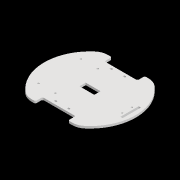
# Autodesk Inventor part: Parte inferior 2 v1
Saved by Autodesk Inventor 2022 (Build 260153000, 153)
## iProperties
Created: 2021-09-27
Part Number: Parte inferior 2 v1
Material: Genérico
Document SubType Name: Modeling
Designer: Julio R
Density: 1 g/cm^3
Appearance: Valor por defecto
Author: Julio R
Autodesk Inventor part; units mm, degrees
ref_plane "YZ Plane" through (0, 0, 0) normal (1, 0, 0) x (0, 1, 0)
ref_plane "XZ Plane" through (0, 0, 0) normal (0, 1, 0) x (-1, 0, 0)
ref_plane "XY Plane" through (0, 0, 0) normal (0, 0, 1) x (1, 0, 0)
sketch "Boceto2" plane through (0, 0, 0) normal (0, 1, 0) x (-1, 0, 0)
  circle A0 centre (0, 0) radius 62.5
  line L0 (15, 32.5) -> (15, -32.5)
  line L1 (15, -32.5) -> (45, -32.5)
  line L2 (45, -32.5) -> (45, 32.5)
  line L3 (45, 32.5) -> (15, 32.5)
  circle A1 centre (18.5, -29) radius 1.25
  line L4 (0, 6.809) -> (0, -6.809)
  line L5 (-6.4675, 0) -> (6.4675, 0) construction
  circle A2 centre (41.5, -29) radius 1.25
  circle A3 centre (18.5, 29) radius 1.25
  circle A4 centre (41.5, 29) radius 1.25
  line L6 (7.5, -42.3) -> (-7.5, -42.3)
  line L7 (-7.5, -42.3) -> (-7.5, -25)
  line L8 (-7.5, -25) -> (7.5, -25)
  line L9 (7.5, -25) -> (7.5, -42.3)
  arc A5 (9, -42.3) -> (9, -33.8) centre (9, -38.05) ccw
  line L10 (9, -42.3) -> (7.5, -42.3)
  line L11 (9, -33.8) -> (7.5, -33.8)
  arc A6 (9.5, -39.2) -> (9.5, -36.9) centre (9.5, -38.05) ccw
  line L12 (9.5, -39.2) -> (7.5, -39.2)
  line L13 (7.5, -39.2) -> (7.5, -36.9)
  line L14 (7.5, -36.9) -> (9.5, -36.9)
  line L15 (9.5, -36.9) -> (9.5, -39.2)
  arc A7 (-9, -33.8) -> (-9, -42.3) centre (-9, -38.05) ccw
  line L16 (-9, -42.3) -> (-7.5, -42.3)
  line L17 (-9, -33.8) -> (-7.5, -33.8)
  arc A8 (-9.5, -36.9) -> (-9.5, -39.2) centre (-9.5, -38.05) ccw
  line L18 (-9.5, -39.2) -> (-7.5, -39.2)
  line L19 (-7.5, -39.2) -> (-7.5, -36.9)
  line L20 (-7.5, -36.9) -> (-9.5, -36.9)
  line L21 (-9.5, -36.9) -> (-9.5, -39.2)
  line L22 (7.5, 42.3) -> (-7.5, 42.3)
  line L23 (-7.5, 42.3) -> (-7.5, 25)
  line L24 (-7.5, 25) -> (7.5, 25)
  line L25 (7.5, 25) -> (7.5, 42.3)
  arc A9 (9, 33.8) -> (9, 42.3) centre (9, 38.05) ccw
  line L26 (9, 42.3) -> (7.5, 42.3)
  line L27 (9, 33.8) -> (7.5, 33.8)
  arc A10 (9.5, 36.9) -> (9.5, 39.2) centre (9.5, 38.05) ccw
  line L28 (9.5, 39.2) -> (7.5, 39.2)
  line L29 (7.5, 39.2) -> (7.5, 36.9)
  line L30 (7.5, 36.9) -> (9.5, 36.9)
  line L31 (9.5, 36.9) -> (9.5, 39.2)
  line L32 (-9, 33.8) -> (-7.5, 33.8)
  line L33 (-7.5, 36.9) -> (-9.5, 36.9)
  line L34 (-7.5, 39.2) -> (-7.5, 36.9)
  line L35 (-9.5, 36.9) -> (-9.5, 39.2)
  line L36 (-9.5, 39.2) -> (-7.5, 39.2)
  arc A11 (-9.5, 39.2) -> (-9.5, 36.9) centre (-9.5, 38.05) ccw
  line L37 (-9, 42.3) -> (-7.5, 42.3)
  arc A12 (-9, 42.3) -> (-9, 33.8) centre (-9, 38.05) ccw
  line L38 (-15, -31) -> (-48, -31)
  line L39 (-48, -31) -> (-48, 31)
  line L40 (-48, 31) -> (-15, 31)
  line L41 (-15, 31) -> (-15, -31)
  line L42 (10.1, -4.25) -> (-10.1, -4.25)
  line L43 (-10.1, -4.25) -> (-10.1, 4.25)
  line L44 (-10.1, 4.25) -> (10.1, 4.25)
  line L45 (10.1, 4.25) -> (10.1, -4.25)
  line L46 (46.0104, -42.3) -> (-46.0104, -42.3)
  line L47 (-46.0104, -42.3) -> (-46.0104, 42.3)
  line L48 (-46.0104, 42.3) -> (46.0104, 42.3)
  line L49 (46.0104, 42.3) -> (46.0104, -42.3)
  line L50 (-54, -12.5) -> (-57, -12.5)
  line L51 (-57, -12.5) -> (-57, 12.5)
  line L52 (-57, 12.5) -> (-54, 12.5)
  line L53 (-54, 12.5) -> (-54, -12.5)
  line L54 (58.7, -12.5) -> (46, -12.5)
  line L55 (46, -12.5) -> (46, 7.82)
  line L56 (46, 7.82) -> (58.7, 7.82)
  line L57 (58.7, 7.82) -> (58.7, -12.5)
  line L58 (22.5, 52.3) -> (-22.5, 52.3)
  line L59 (-22.5, 52.3) -> (-22.5, 42.3)
  line L60 (-22.5, 42.3) -> (22.5, 42.3)
  line L61 (22.5, 42.3) -> (22.5, 52.3)
  line L62 (22.5, -52.3) -> (-22.5, -52.3)
  line L63 (-22.5, -52.3) -> (-22.5, -42.3)
  line L64 (-22.5, -42.3) -> (22.5, -42.3)
  line L65 (22.5, -42.3) -> (22.5, -52.3)
  line L66 (22.5, 52.3) -> (34.2193, 52.3)
  line L67 (-22.5, 52.3) -> (-34.2193, 52.3)
  line L68 (22.5, -52.3) -> (34.2193, -52.3)
  line L69 (-22.5, -52.3) -> (-34.2193, -52.3)
  circle A13 centre (-50.6, 6.809) radius 1.15
  circle A14 centre (-50.6, -6.653) radius 1.15
  point P0 (45, 0)
  point P1 (13.25, -38.05)
  point P2 (10.65, -38.05)
  point P3 (-13.25, -38.05)
  point P4 (-10.65, -38.05)
  point P5 (13.25, 38.05)
  point P6 (10.65, 38.05)
  point P7 (-10.65, 38.05)
  point P8 (-13.25, 38.05)
  point P9 (-15, 0)
  point P10 (0, -4.25)
  point P11 (10.1, 0)
  point P12 (-54, 0)
  point P13 (9, 42.3)
  point P14 (0, 52.3)
  point P15 (-22.5, -42.3)
  point P16 (22.5, -42.3)
  point P17 (22.5, 42.3)
  dimension "d51" = 125
  dimension "d52" = 65
  dimension "d53" = 30
  dimension "d56" = 3.5
  dimension "d57" = 3.5
  dimension "d60" = 23
  dimension "d63" = 58
  dimension "d70" = 15
  dimension "d78" = 15
  dimension "d79" = 17.3
  dimension "d80" = 8.5
  dimension "d81" = 1.5
  dimension "d82" = 4.25
  dimension "d83" = 1.15
  dimension "d84" = 2.3
  dimension "d86" = 2
  dimension "d87" = 25
  dimension "d88" = 7.5
  dimension "d89" = 33
  dimension "d90" = 62
  dimension "d91" = 15
  dimension "d92" = 20.2
  dimension "d93" = 8.5
  dimension "d94" = 3
  dimension "d95" = 25
  dimension "d98" = 6
  dimension "d99" = 12.7
  dimension "d100" = 20.32
  dimension "d101" = 1
  dimension "d102" = 20
  dimension "d108" = 10
  dimension "d113" = 45
  dimension "d114" = 13.462
  dimension "d115" = 3.4
  dimension "d116" = 2.3
  dimension "d119" = 2.3
  constraints: 140 end point, 41 symmetric about line, 24 point on circle, 20 parallel, 15 centre point, 13 horizontal, 9 perpendicular, 8 midpoint, 5 horizontal alignment, 4 coincident, 4 collinear, 4 point on line, 4 vertical alignment, 2 vertical, 12 other
  measures "d51" diameter of A0
  measures "d52" distance of L2.end L1.end
  measures "d53" distance of L1.end L0.end
  measures "d56" horizontal distance of A1.centre L0.end
  measures "d57" horizontal distance of L0.end A1.centre
  measures "d60" distance of A1.centre A2.centre
  measures "d63" distance of A1.centre A3.centre
  measures "d70" distance from line of point (0, 0) L0
  measures "d78" distance of L7.end L8.end
  measures "d79" distance of L6.end L7.end
  measures "d80" distance between parallel lines of L11 L10
  measures "d81" distance from line of L9 A5.centre
  measures "d82" radius of A5
  measures "d83" radius of A6
  measures "d84" distance between parallel lines of L14 L12
  measures "d86" distance from line of L13 A6.centre
  measures "d87" distance from line of point (0, 0) L8
  measures "d88" distance from line of point (0, 0) L9
  measures "d89" distance of L39.end L40.end
  measures "d90" distance of L38.end L39.end
  measures "d91" distance from line of point (0, 0) L41
  measures "d92" distance of L43.end L44.end
  measures "d93" distance of L42.end L43.end
  measures "d94" distance between parallel lines of L51 L53
  measures "d95" distance between parallel lines of L52 L50
  measures "d98" distance between parallel lines of L39 L53
  measures "d99" distance of L55.end L56.end
  measures "d100" distance of L54.end L55.end
  measures "d101" distance between parallel lines of L2 L55
  measures "d102" distance between parallel lines of L1 L54
  measures "d108" distance of L59.end L58.end
  measures "d113" distance between parallel lines of L59 L61
  measures "d114" distance of A14.centre A13.centre
  measures "d115" distance from line of L53 A13.centre
  measures "d116" diameter of A13
  measures "d119" diameter of A14
extrude "Extrusión4" add sketch "Boceto2" along normal blind 3 contours A0 L49 L54 L57 L56 | L48 L61 L66 A0 | L49 L56 L55 L54 L46 A5 L11 L9 L8 L7 L17 A7 L47 L38 L41 L40 L48 A12 L32 L23 L24 L25 L27 A9 | A0 L68 L65 L46 | L66 L58 L67 A0 | L48 L26 L22 L37 L59 L58 L61 | L56 L57 L54 L49 | L49 L54 L55 L56 | A0 L69 L62 L68 | L65 L62 L63 L46 L16 L6 L10 | L67 L59 L48 A0 | A9 L27 L25 L30 A10 L28 L26 | A0 L46 L63 L69 | L10 L9 L12 A6 L14 L11 A5 | L47 L40 L39 L38 A0 | L25 L24 L23 L22 | L6 L7 L8 L9 | L47 L38 L39 L40 | L40 L41 L38 L47 | L23 L36 A11 L33 L32 A12 L37 | L28 L31 L30 L25 | L16 A7 L17 L7 L20 A8 L18 | L9 L14 L15 L12 | L23 L33 L35 L36 | A10 L31 | L18 L21 L20 L7 | L15 A6 | L35 A11 | A8 L21 | L3 L2 L1 L0 | A1 | L44 L45 L42 L4 | L4 L42 L43 L44 | A2 | A3 | A4 | L50 L51 L52 L53 | A13 | A14
extrude "Extrusión5" cut sketch "Boceto2" along normal blind 3 contours L48 L61 L66 A0 | A0 L68 L65 L46 | L66 L58 L67 A0 | L48 L26 L22 L37 L59 L58 L61 | A0 L69 L62 L68 | L65 L62 L63 L46 L16 L6 L10 | L67 L59 L48 A0 | A0 L46 L63 L69 | L28 L31 L30 L25 | L9 L14 L15 L12 | L23 L33 L35 L36 | A10 L31 | L18 L21 L20 L7 | L15 A6 | L35 A11 | A8 L21 | A1 | L44 L45 L42 L4 | L4 L42 L43 L44 | A2 | A3 | A4 | L50 L51 L52 L53
extrude "Extrusión6" add sketch "Boceto2" along normal blind 3 contours L48 L61 L66 A0 | A0 L68 L65 L46 | L67 L59 L48 A0 | A0 L46 L63 L69
fillet "Empalme3" radius 2 8 edges at (-22.5, 1.5, -42.3) (-22.5, 1.5, -52.3) (22.5, 1.5, -42.3) (22.5, 1.5, -52.3) (-22.5, 1.5, 52.3) (-22.5, 1.5, 42.3) (22.5, 1.5, 42.3) (22.5, 1.5, 52.3)
fillet "Empalme4" radius 20 4 edges at (-34.2193, 1.5, 52.3) (34.2193, 1.5, 52.3) (-34.2193, 1.5, -52.3) (34.2193, 1.5, -52.3)
extrude "Extrusión7" cut sketch "Boceto2" along normal blind 3 contours A13 | A14
